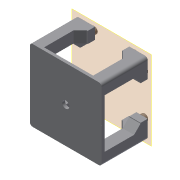
# Autodesk Inventor part: 30_IM_LED_holder_forcube_v3
Saved by Autodesk Inventor 2019.4 (Build 234330000, 330)
## iProperties
Created: 2021-01-15
Part Number: 30_IM_LED_holder_forcube_v3
Material: Generic
Document SubType Name: Modeling
Designer: diederichbenedict
Density: 1 g/cm^3
Appearance: Default
Author: diederichbenedict
Autodesk Inventor part; units mm, degrees
ref_plane "YZ Plane" through (0, 0, 0) normal (1, 0, 0) x (0, 1, 0)
ref_plane "XZ Plane" through (0, 0, 0) normal (0, 1, 0) x (-1, 0, 0)
ref_plane "XY Plane" through (0, 0, 0) normal (0, 0, 1) x (1, 0, 0)
ref_plane "Work Plane1" through (0, 0, 0) normal (0, 0, 1) x (1, 0, 0)
sketch "Sketch1" plane through (0, 0, 0) normal (0, 0, 1) x (1, 0, 0)
  circle A0 centre (21, -21) radius 1.65 construction
  circle A1 centre (-21, 21) radius 1.65 construction
  circle A2 centre (21, 21) radius 1.65 construction
  circle A3 centre (-21, -21) radius 1.65 construction
  arc A4 (23, -25) -> (25, -23) centre (23, -23) ccw construction
  line L0 (25, -23) -> (25, 23) construction
  arc A5 (25, 23) -> (23, 25) centre (23, 23) ccw construction
  line L1 (23, 25) -> (-23, 25) construction
  arc A6 (-23, 25) -> (-25, 23) centre (-23, 23) ccw construction
  line L2 (-25, 23) -> (-25, -23) construction
  arc A7 (-25, -23) -> (-23, -25) centre (-23, -23) ccw construction
  line L3 (-23, -25) -> (23, -25) construction
  circle A8 centre (0, 0) radius 16 construction
  circle A9 centre (14.5, 20.8) radius 2.65 construction
  circle A10 centre (-14.5, 20.8) radius 2.65 construction
  circle A11 centre (14.5, -20.8) radius 2.65 construction
  circle A12 centre (20.8, 14.5) radius 2.65 construction
  circle A13 centre (20.8, -14.5) radius 2.65 construction
  circle A14 centre (-20.8, 14.5) radius 2.65 construction
  circle A15 centre (-14.5, -20.8) radius 2.65 construction
  circle A16 centre (-20.8, -14.5) radius 2.65 construction
  circle A17 centre (0.2, -0.14) radius 10.16 construction
  circle A18 centre (21, -21) radius 1.65 construction
  circle A19 centre (-21, 21) radius 1.65 construction
  circle A20 centre (21, 21) radius 1.65 construction
  circle A21 centre (-21, -21) radius 1.65 construction
  arc A22 (23, -25) -> (25, -23) centre (23, -23) ccw construction
  line L4 (25, -23) -> (25, 23) construction
  arc A23 (25, 23) -> (23, 25) centre (23, 23) ccw construction
  line L5 (23, 25) -> (-23, 25) construction
  arc A24 (-23, 25) -> (-25, 23) centre (-23, 23) ccw construction
  line L6 (-25, 23) -> (-25, -23) construction
  arc A25 (-25, -23) -> (-23, -25) centre (-23, -23) ccw construction
  line L7 (-23, -25) -> (23, -25) construction
  circle A26 centre (0, 0) radius 16 construction
  circle A27 centre (14.5, 20.8) radius 2.65 construction
  circle A28 centre (-14.5, 20.8) radius 2.65 construction
  circle A29 centre (14.5, -20.8) radius 2.65 construction
  circle A30 centre (20.8, 14.5) radius 2.65 construction
  circle A31 centre (20.8, -14.5) radius 2.65 construction
  circle A32 centre (-20.8, 14.5) radius 2.65 construction
  circle A33 centre (-14.5, -20.8) radius 2.65 construction
  circle A34 centre (-20.8, -14.5) radius 2.65 construction
  line L8 (-24.65, 22.71) -> (-24.65, -22.99) construction
  line L9 (-16.77, -17.11) -> (-16.77, 16.83) construction
  line L10 (-16.77, -17.11) -> (-16.77, 16.83) construction
  line L11 (17.17, -17.11) -> (-16.77, -17.11) construction
  line L12 (17.17, -17.11) -> (-16.77, -17.11) construction
  line L13 (0, -25) -> (0, -17.11) construction
  arc A35 (-24.65, -22.99) -> (-22.65, -24.99) centre (-22.65, -22.99) ccw construction
  line L14 (-16.77, 0) -> (-24.65, 0) construction
  line L15 (-24.65, -0.14) -> (-16.77, -0.14)
  line L16 (-16.77, -0.14) -> (-16.77, -25)
  line L17 (-16.77, -25) -> (-22.65, -25)
  line L18 (-24.65, -23) -> (-24.65, -0.14)
  line L19 (-16.77, -25) -> (0.2, -25)
  line L20 (0.2, -25) -> (0.2, -17.11)
  line L21 (0.2, -17.11) -> (-16.77, -17.11)
  line L22 (-16.77, -17.11) -> (-16.77, -25)
  arc A36 (-24.65, -23) -> (-22.65, -25) centre (-22.65, -23) ccw
  line L23 (-16.77, -11.85) -> (-24.65, -11.85)
  line L24 (-11.85, -17.11) -> (-11.85, -25)
  dimension "d1" = 2
  constraints: 24 end point, 8 point on line, 6 perpendicular, 4 parallel, 4 tangent, 3 midpoint, 2 horizontal, 2 point on circle, 1 centre point
  measures "d1" radius of A36
extrude "Extrusion1" add sketch "Sketch1" along normal blind 5 contours L23 L16 L17 A36 L18 | L21 L24 L19 L16
sketch "Sketch2" plane through (0, 0, 0) normal (0, 0, -1) x (-1, 0, 0)
  circle A0 centre (20.46, -14.44) radius 2.475 projected
  circle A1 centre (14.1, -20.8) radius 2.475 projected
  point P0 (0, 0)
extrude "Extrusion2" add sketch "Sketch2" along normal blind 2 draft -2
sketch "Sketch3" plane through (0, 0, 5) normal (0, 0, 1) x (1, 0, 0)
  line L0 (-22.65, -25) -> (-11.85, -25) projected
  line L1 (-11.85, -25) -> (-11.85, -17.11) projected
  line L2 (-11.85, -17.11) -> (-16.77, -17.11) projected
  line L3 (-16.77, -17.11) -> (-16.77, -11.85) projected
  line L4 (-16.77, -11.85) -> (-24.65, -11.85) projected
  line L5 (-24.65, -11.85) -> (-24.65, -23) projected
  arc A0 (-24.65, -23) -> (-22.65, -25) centre (-22.65, -23) ccw projected
  line L6 (-11.85, -17.11) -> (-16.77, -17.11) projected
  line L7 (-16.77, -17.11) -> (-24.65, -17.11)
  line L8 (-16.77, -17.11) -> (-16.77, -25)
  line L9 (-22.65, -25) -> (-11.85, -25) projected
  point P0 (0, 0)
  constraints: 4 end point, 2 point on line, 1 collinear, 1 perpendicular
extrude "Extrusion3" add sketch "Sketch3" along normal blind 25 contours A0 L5 L7 L8 L0
chamfer "Chamfer1" distance 4.5 angle 45 2 edges at (-16.77, -21.055, 5) (-20.71, -17.11, 5)
sketch "Sketch4" plane through (0, 0, 30) normal (0, 0, 1) x (1, 0, 0)
  line L0 (-22.65, -25) -> (-16.77, -25) projected
  line L1 (-16.77, -25) -> (-16.77, -17.11) projected
  line L2 (-16.77, -17.11) -> (-24.65, -17.11) projected
  line L3 (-24.65, -17.11) -> (-24.65, -23) projected
  arc A0 (-24.65, -23) -> (-22.65, -25) centre (-22.65, -23) ccw projected
  line L4 (-24.65, -17.11) -> (-24.65, 0)
  line L5 (0.2, -0.14) -> (0.2, -25)
  line L6 (0.2, -25) -> (-16.77, -25)
  line L7 (-22.65, -25) -> (-11.85, -25) projected
  line L8 (-34.59, -0.14) -> (34.99, -0.14)
  line L9 (-24.65, -0.14) -> (0.2, -0.14)
  point P0 (0, 0)
  constraints: 10 end point, 3 point on line, 2 midpoint, 1 collinear, 1 horizontal, 1 vertical, 2 other
extrude "Extrusion4" add sketch "Sketch4" along normal blind 2
pattern_circular "Circular Pattern1" count 4 over 360 about axis through (0.2, -0.14, 30) along (0, 0, 1) of "Extrusion1", "Extrusion2", "Extrusion3", "Chamfer1", "Extrusion4"
sketch "Sketch5" plane through (0, 0, 32) normal (0, 0, 1) x (1, 0, 0)
  circle A0 centre (0.2, -0.14) radius 10.16 projected
  circle A1 centre (0.2, -0.14) radius 2.5
  point P0 (0, 0)
  dimension "d18" = 5
  constraints: 1 centre point, 1 coincident
  measures "d18" diameter of A1
extrude "Extrusion5" cut sketch "Sketch5" against normal blind 2 contours A1
body "Solid1"
